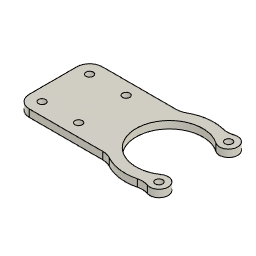
uWAVE_holder_flat (Autodesk Fusion 360 design; units mm, degrees)
Autodesk Fusion 360 part; units mm, degrees
sketch "Sketch1" plane through (0, 0, 0) normal (0, 0, 1) x (1, 0, 0)
  circle A0 centre (13.3357, 19.0453) radius 5
  circle A1 centre (13.3357, -19.0453) radius 5
  line L0 (0, 0) -> (80.5902, 0) construction
  line L1 (0, 0) -> (13.3357, 19.0453) construction
  arc A2 (10.4678, 14.9495) -> (10.4678, -14.9495) centre (0, 0) ccw
  arc A3 (9.5367, 22.2961) -> (9.5367, -22.2961) centre (0, 0) ccw
  line L2 (-13.7136, 20) -> (-56.7136, 20)
  line L3 (-56.7136, -20) -> (-13.7136, -20)
  line L4 (0, 0) -> (-230.6085, 0) construction
  circle A4 centre (13.3357, 19.0453) radius 2
  circle A5 centre (13.3357, -19.0453) radius 2
  line L5 (-63.7136, 13) -> (-63.7136, -13)
  arc A6 (-56.7136, 20) -> (-63.7136, 13) centre (-56.7136, 13) ccw
  arc A7 (-63.7136, -13) -> (-56.7136, -20) centre (-56.7136, -13) ccw
  circle A8 centre (-56.7136, 13) radius 2
  circle A9 centre (-56.7136, -13) radius 2
  circle A10 centre (-36.7136, 13) radius 2
  circle A11 centre (-36.7136, -13) radius 2
  point P0 (-63.7136, 20)
  point P1 (-63.7136, -20)
  dimension "d1" = 36.5
  dimension "d2" = 6
  dimension "d3" = 55
  dimension "d4" = 10
  dimension "d5" = 40
  dimension "d23" = 4
  dimension "d25" = 50
  dimension "d26" = 7
  dimension "d27" = 4
  dimension "d30" = 20
  constraint coincident L0.start L1.start
  constraint tangent A0 A2
  constraint tangent A1 A2
  constraint horizontal L0
  constraint coincident A0.centre L1.end
  constraint symmetric A0.centre A1.centre L0
  constraint coincident A0 A2.start
  constraint coincident A1 A2.end
  constraint coincident A0 A3.start
  constraint coincident A1 A3.end
  constraint coincident A3 L2.start
  constraint coincident A3 L3.end
  constraint concentric A0 A4
  constraint concentric A1 A5
  constraint equal A4 A5
  constraint horizontal L2
  constraint perpendicular L2 L5
  constraint perpendicular L3 L5
  constraint coincident P0 L2
  constraint coincident P0 L5
  constraint tangent L2 A6
  constraint tangent L5 A6
  constraint coincident P1 L3
  constraint coincident P1 L5
  constraint tangent L3 A7
  constraint tangent L5 A7
  constraint equal A6 A7
  constraint concentric A6 A8
  constraint concentric A7 A9
  constraint equal A10 A11
  constraint equal A8 A10
  constraint symmetric L4 A10.centre A11.centre
  constraint horizontal A6.centre A10.centre
  constraint equal A8 A9
  constraint symmetric L2 L3 L4
  measures "d1" diameter of A2
  measures "d2" distance of A2 A3
  measures "d3" angle of L0 L1
  measures "d4" diameter of A0
  measures "d5" distance of P0 P1
  measures "d23" diameter of A4
  measures "d25" distance of L2.start P0
  measures "d26" radius of A6
  measures "d27" diameter of A8
  measures "d30" horizontal distance of A6.centre A10.centre
extrude "Extrude1" add sketch "Sketch1" along normal blind 4
fillet "Fillet1" radius 10 4 edges at (9.5367, 22.2961, 2) (-13.7136, 20, 2) (9.5367, -22.2961, 2) (-13.7136, -20, 2)
